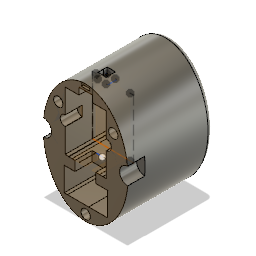
Magnets_Design v1 (Autodesk Fusion 360 design; units mm, degrees)
Autodesk Fusion 360 part; units mm, degrees
note: some values were not read from the file. Set by a fixed rule: which sketch regions a step uses.
(part 1 of 2)
sketch "Sketch1" plane through (0, 0, 0) normal (0, 0, 1) x (1, 0, 0)
  ellipse E0 centre (0, 0) end of major axis (0, 44.45) minor radius 31.75
  line L0 (0, -44.45) -> (0, 44.45)
  line L1 (31.75, 0) -> (-31.75, 0)
extrude "Extrude1" add sketch "Sketch1" along normal blind 63.5
sketch "Sketch2" plane through (0, 0, 63.5) normal (0, 0, 1) x (1, 0, 0)
  ellipse E0 centre (0, 0) end of major axis (0, 44.45) minor radius 31.75
  line L0 (0.1301, 25.8411) -> (10.2901, 25.8411)
  line L1 (0.1301, 25.8411) -> (-10.0299, 25.8411)
  line L2 (-10.0299, 34.8417) -> (-10.0299, -8.8463)
  line L3 (-10.0299, 34.8417) -> (10.4165, 34.8417)
  line L4 (10.4165, 34.8417) -> (10.4165, -8.8757)
  line L5 (10.4165, -8.8757) -> (-10.0299, -8.8463)
  line L6 (0.1933, 34.8417) -> (5.2733, 34.8417)
  line L7 (0.1933, 34.8417) -> (-4.8867, 34.8417)
  line L8 (-4.8867, 34.8417) -> (-4.8867, 39.9217)
  line L9 (-4.8867, 39.9217) -> (5.2733, 39.9217)
  line L10 (5.2733, 39.9217) -> (5.2733, 34.8417)
  dimension "d3" = 10.16
  dimension "d4" = 10.16
  dimension "d5" = 43.688
  dimension "d6" = 5.08
  dimension "d7" = 5.08
  dimension "d8" = 5.08
  measures "d3" distance of E0.centre
  measures "d4" distance of E0.centre
  measures "d6" distance of E0.centre
  measures "d7" distance of E0.centre
extrude "Extrude2" cut sketch "Sketch2" against normal blind 17.78 contours L2 L3 L4 L5 L6 L7 | L3 L6 L7 L8 L9 L10
extrude "Extrude3" cut 1 faces at (1.8866, 5.7066, 45.72) along direction (0, 0, -1) blind 2.54
sketch "Sketch3" plane through (0, 0, 63.5) normal (0, 0, 1) x (1, 0, 0)
  line L0 (10.4165, -8.8757) -> (-10.0299, -8.8463)
  line L1 (-10.0299, -8.8463) -> (-10.0299, 34.8417)
  line L2 (-10.0299, 34.8417) -> (-4.8867, 34.8417)
  line L3 (-4.8867, 34.8417) -> (-4.8867, 39.9217)
  line L4 (-4.8867, 39.9217) -> (5.2733, 39.9217)
  line L5 (5.2733, 39.9217) -> (5.2733, 34.8417)
  line L6 (5.2733, 34.8417) -> (10.4165, 34.8417)
  line L7 (10.4165, 34.8417) -> (10.4165, -8.8757)
  ellipse E0 centre (0, 0) end of major axis (0, 44.45) minor radius 31.75
  line L8 (0.1933, -16.0726) -> (13.7823, -16.0922)
  line L9 (0.1933, -16.0726) -> (-13.3957, -16.053)
  line L10 (13.7823, -16.0922) -> (13.7567, -33.8722)
  line L11 (-13.3957, -16.053) -> (-13.4213, -33.833)
  line L12 (-13.4213, -33.833) -> (13.7567, -33.8722)
  dimension "d13" = 13.589
  dimension "d14" = 13.589
  dimension "d15" = 17.78
  dimension "d16" = 17.78
extrude "Extrude4" cut sketch "Sketch3" against normal blind 53.34 contours L8 L9 L10 L11 L12
sketch "Sketch4" plane through (0, 0, 63.5) normal (0, 0, 1) x (1, 0, 0)
  line L0 (-13.4213, -33.833) -> (-13.3957, -16.053)
  line L1 (-13.3957, -16.053) -> (13.7823, -16.0922)
  line L2 (13.7823, -16.0922) -> (13.7567, -33.8722)
  line L3 (13.7567, -33.8722) -> (-13.4213, -33.833)
  line L4 (10.4165, -8.8757) -> (-10.0299, -8.8463)
  line L5 (-10.0299, -8.8463) -> (-10.0299, 34.8417)
  line L6 (-10.0299, 34.8417) -> (-4.8867, 34.8417)
  line L7 (-4.8867, 34.8417) -> (-4.8867, 39.9217)
  line L8 (-4.8867, 39.9217) -> (5.2733, 39.9217)
  line L9 (5.2733, 39.9217) -> (5.2733, 34.8417)
  line L10 (5.2733, 34.8417) -> (10.4165, 34.8417)
  line L11 (10.4165, 34.8417) -> (10.4165, -8.8757)
  ellipse E0 centre (0, 0) end of major axis (0, 44.45) minor radius 31.75
  line L12 (-4.5003, -8.861) -> (-4.5107, -16.0658)
  line L13 (4.8218, -8.861) -> (4.8114, -16.0792)
  line L14 (-4.5003, -8.861) -> (4.8218, -8.861)
  line L15 (4.8114, -16.0792) -> (-4.5107, -16.0658)
extrude "Extrude5" cut sketch "Sketch4" against normal blind 12.7 contours L1 L4 L12 L13 L14 L15
sketch "Sketch5" plane through (0, 0, 63.5) normal (0, 0, 1) x (1, 0, 0)
  ellipse E0 centre (0, 0) end of major axis (0, 44.45) minor radius 31.75
  line L0 (-4.5107, -16.0658) -> (-4.5003, -8.861)
  line L1 (-4.5003, -8.861) -> (0.1933, -8.861)
  line L2 (0.1933, -8.861) -> (-10.0299, -8.8463)
  line L3 (-10.0299, -8.8463) -> (-10.0299, 34.8417)
  line L4 (-10.0299, 34.8417) -> (-4.8867, 34.8417)
  line L5 (-4.8867, 34.8417) -> (-4.8867, 39.9217)
  line L6 (-4.8867, 39.9217) -> (5.2733, 39.9217)
  line L7 (5.2733, 39.9217) -> (5.2733, 34.8417)
  line L8 (5.2733, 34.8417) -> (10.4165, 34.8417)
  line L9 (10.4165, 34.8417) -> (10.4165, -8.8757)
  line L10 (10.4165, -8.8757) -> (4.8218, -8.8677)
  line L11 (4.8218, -8.8677) -> (4.8114, -16.0792)
  line L12 (4.8114, -16.0792) -> (13.7823, -16.0922)
  line L13 (13.7823, -16.0922) -> (13.7567, -33.8722)
  line L14 (13.7567, -33.8722) -> (-13.4213, -33.833)
  line L15 (-13.4213, -33.833) -> (-13.3957, -16.053)
  line L16 (-13.3957, -16.053) -> (-4.5107, -16.0658)
  circle A0 centre (31.7466, 0.6522) radius 6.35
  circle A1 centre (-31.7467, 0.6454) radius 6.35
  circle A2 centre (-10.0299, 12.9977) radius 6.35
  circle A3 centre (10.4165, 12.983) radius 6.35
  dimension "d21" = 12.7
  dimension "d22" = 12.7
  dimension "d23" = 12.7
  dimension "d24" = 12.7
  measures "d21" diameter of A0
  measures "d22" diameter of A1
  measures "d23" diameter of A2
  measures "d24" diameter of A3
extrude "Extrude6" cut sketch "Sketch5" against normal blind 12.7 contours E0 A1 | E0 A0 | L3 A2 | L9 A3 picked at (-29.7962, -0.9171) picked at (29.729, 2.0886) picked at (-11.8462, 11.3429) picked at (12.7487, 12.3651)
sketch "Sketch6" plane through (0, 0, 63.5) normal (0, 0, 1) x (1, 0, 0)
  arc A0 (-31.4879, -5.6993) -> (-31.3557, 6.9834) centre (-31.7467, 0.6454) ccw
  ellipse E0 centre (0, 0) end of major axis (0, 44.45) minor radius 31.75 (-31.4879, -5.6993) -> (31.4886, -5.6926) ccw
  arc A1 (31.355, 6.9901) -> (31.4886, -5.6926) centre (31.7466, 0.6522) ccw
  ellipse E1 centre (0, 0) end of major axis (0, 44.45) minor radius 31.75 (31.355, 6.9901) -> (-31.3557, 6.9834) ccw
  arc A2 (-10.0299, 19.3477) -> (-10.0299, 6.6477) centre (-10.0299, 12.9977) ccw
  line L0 (-10.0299, 19.3477) -> (-10.0299, 34.8417)
  line L1 (-10.0299, 34.8417) -> (-4.8867, 34.8417)
  line L2 (-4.8867, 34.8417) -> (-4.8867, 39.9217)
  line L3 (-4.8867, 39.9217) -> (5.2733, 39.9217)
  line L4 (5.2733, 39.9217) -> (5.2733, 34.8417)
  line L5 (5.2733, 34.8417) -> (10.4165, 34.8417)
  line L6 (10.4165, 34.8417) -> (10.4165, 19.333)
  arc A3 (10.4165, 6.633) -> (10.4165, 19.333) centre (10.4165, 12.983) ccw
  line L7 (10.4165, 6.633) -> (10.4165, -8.8757)
  line L8 (10.4165, -8.8757) -> (4.8218, -8.8677)
  line L9 (4.8218, -8.8677) -> (4.8114, -16.0792)
  line L10 (4.8114, -16.0792) -> (13.7823, -16.0922)
  line L11 (13.7823, -16.0922) -> (13.7567, -33.8722)
  line L12 (13.7567, -33.8722) -> (-13.4213, -33.833)
  line L13 (-13.4213, -33.833) -> (-13.3957, -16.053)
  line L14 (-13.3957, -16.053) -> (-4.5107, -16.0658)
  line L15 (-4.5107, -16.0658) -> (-4.5003, -8.861)
  line L16 (-4.5003, -8.861) -> (0.1933, -8.861)
  line L17 (0.1933, -8.861) -> (-10.0299, -8.8463)
  line L18 (-10.0299, -8.8463) -> (-10.0299, 6.6477)
  line L19 (22.8671, 20.3792) -> (17.7871, 20.3792)
  line L20 (17.7871, 20.3792) -> (17.7871, 25.4592)
  line L21 (17.7871, 25.4592) -> (22.8671, 25.4592)
  line L22 (22.8671, 25.4592) -> (22.8671, 20.3792)
  line L23 (22.8671, 20.3792) -> (17.7871, 25.4592) construction
  line L24 (17.7871, 20.3792) -> (22.8671, 25.4592) construction
  line L25 (2.5315, -40.6814) -> (-2.5485, -40.6814)
  line L26 (-2.5485, -40.6814) -> (-2.5485, -35.3439)
  line L27 (-2.5485, -35.3439) -> (2.5315, -35.3439)
  line L28 (2.5315, -35.3439) -> (2.5315, -40.6814)
  line L29 (2.5315, -40.6814) -> (-2.5485, -35.3439) construction
  line L30 (-2.5485, -40.6814) -> (2.5315, -35.3439) construction
  line L31 (-17.6615, 20.3792) -> (-22.7415, 20.3792)
  line L32 (-22.7415, 20.3792) -> (-22.7415, 25.4592)
  line L33 (-22.7415, 25.4592) -> (-17.6615, 25.4592)
  line L34 (-17.6615, 25.4592) -> (-17.6615, 20.3792)
  line L35 (-17.6615, 20.3792) -> (-22.7415, 25.4592) construction
  line L36 (-22.7415, 20.3792) -> (-17.6615, 25.4592) construction
  dimension "d27" = 5.08
  dimension "d28" = 5.08
  dimension "d30" = 5.08
  dimension "d31" = 5.08
  dimension "d32" = 5.08
  measures "d28" distance of E0.centre
  measures "d31" distance of E0.centre
extrude "Extrude7" cut sketch "Sketch6" against normal blind 5.08 contours L19 L20 L21 L22 | L25 L26 L27 L28 | L31 L32 L33 L34
sketch "Sketch7" plane through (0, 0, 63.5) normal (0, 0, 1) x (1, 0, 0)
  line L0 (17.7871, 20.3792) -> (17.7871, 25.4592)
  line L1 (17.7871, 25.4592) -> (22.8671, 25.4592)
  line L2 (22.8671, 25.4592) -> (22.8671, 20.3792)
  line L3 (22.8671, 20.3792) -> (17.7871, 20.3792)
  line L4 (-2.5485, -40.6814) -> (-2.5485, -35.3439)
  line L5 (-2.5485, -35.3439) -> (2.5315, -35.3439)
  line L6 (2.5315, -35.3439) -> (2.5315, -40.6814)
  line L7 (2.5315, -40.6814) -> (-2.5485, -40.6814)
  line L8 (-22.7415, 20.3792) -> (-22.7415, 25.4592)
  line L9 (-22.7415, 25.4592) -> (-17.6615, 25.4592)
  line L10 (-17.6615, 25.4592) -> (-17.6615, 20.3792)
  line L11 (-17.6615, 20.3792) -> (-22.7415, 20.3792)
  arc A0 (-31.4879, -5.6993) -> (-31.3557, 6.9834) centre (-31.7467, 0.6454) ccw
  ellipse E0 centre (0, 0) end of major axis (0, 44.45) minor radius 31.75 (-31.4879, -5.6993) -> (31.4886, -5.6926) ccw
  arc A1 (31.355, 6.9901) -> (31.4886, -5.6926) centre (31.7466, 0.6522) ccw
  ellipse E1 centre (0, 0) end of major axis (0, 44.45) minor radius 31.75 (31.355, 6.9901) -> (-31.3557, 6.9834) ccw
  arc A2 (-10.0299, 19.3477) -> (-10.0299, 6.6477) centre (-10.0299, 12.9977) ccw
  line L12 (-10.0299, 19.3477) -> (-10.0299, 34.8417)
  line L13 (-10.0299, 34.8417) -> (-4.8867, 34.8417)
  line L14 (-4.8867, 34.8417) -> (-4.8867, 39.9217)
  line L15 (-4.8867, 39.9217) -> (5.2733, 39.9217)
  line L16 (5.2733, 39.9217) -> (5.2733, 34.8417)
  line L17 (5.2733, 34.8417) -> (10.4165, 34.8417)
  line L18 (10.4165, 34.8417) -> (10.4165, 19.333)
  arc A3 (10.4165, 6.633) -> (10.4165, 19.333) centre (10.4165, 12.983) ccw
  line L19 (10.4165, 6.633) -> (10.4165, -8.8757)
  line L20 (10.4165, -8.8757) -> (4.8218, -8.8677)
  line L21 (4.8218, -8.8677) -> (4.8114, -16.0792)
  line L22 (4.8114, -16.0792) -> (13.7823, -16.0922)
  line L23 (13.7823, -16.0922) -> (13.7567, -33.8722)
  line L24 (13.7567, -33.8722) -> (-13.4213, -33.833)
  line L25 (-13.4213, -33.833) -> (-13.3957, -16.053)
  line L26 (-13.3957, -16.053) -> (-4.5107, -16.0658)
  line L27 (-4.5107, -16.0658) -> (-4.5003, -8.861)
  line L28 (-4.5003, -8.861) -> (0.1933, -8.861)
  line L29 (0.1933, -8.861) -> (-10.0299, -8.8463)
  line L30 (-10.0299, -8.8463) -> (-10.0299, 6.6477)
  line L31 (10.4165, 34.8417) -> (12.9565, 34.8417)
  line L32 (-10.0299, 34.8417) -> (-12.5699, 34.8417)
  line L33 (-12.5699, 34.8417) -> (-12.5699, -8.9534)
  line L34 (-12.5699, -8.9534) -> (-10.0299, -8.8463)
  line L35 (12.9565, 34.8417) -> (12.9565, -8.992)
  line L36 (12.9565, -8.992) -> (10.4165, -8.8757)
  dimension "d36" = 2.54
  dimension "d37" = 2.54
extrude "Extrude8" cut sketch "Sketch7" against normal blind 20.32 contours A2 L12 L32 L33 | A2 L30 L33 L34 | L18 A3 L31 L35 | A3 L19 L35 L36
fillet "Fillet1" radius 3.81 1 edges at (0, -44.45, 0)
sketch "Sketch8" plane through (0, 0, 50.8) normal (0, 0, 1) x (1, 0, 0)
  line L0 (-10.0299, 6.6477) -> (-10.0299, 19.3477)
  arc A0 (-10.0299, 19.3477) -> (-12.5699, 18.8176) centre (-10.0299, 12.9977) ccw
  arc A1 (-12.5699, 18.8176) -> (-12.5699, 7.1778) centre (-10.0299, 12.9977) ccw
  arc A2 (-12.5699, 7.1778) -> (-10.0299, 6.6477) centre (-10.0299, 12.9977) ccw
  line L1 (-12.5699, 18.8176) -> (-12.5699, 7.1778)
  line L2 (12.9565, 18.8029) -> (12.9565, 7.1631)
  line L3 (12.9565, 18.8029) -> (12.9565, 7.1631)
extrude "Extrude9" cut sketch "Sketch8" against normal blind 7.62 contours L0 A0 A2 L1
sketch "Sketch9" plane through (0, 0, 50.8) normal (0, 0, 1) x (1, 0, 0)
  arc A0 (12.9565, 18.8029) -> (10.4165, 19.333) centre (10.4165, 12.983) ccw
  line L0 (10.4165, 19.333) -> (10.4165, 6.633)
  arc A1 (10.4165, 6.633) -> (12.9565, 7.1631) centre (10.4165, 12.983) ccw
  arc A2 (12.9565, 7.1631) -> (12.9565, 18.8029) centre (10.4165, 12.983) ccw
  line L1 (12.9565, 18.8029) -> (12.9565, 7.1631)
extrude "Extrude10" cut sketch "Sketch9" against normal blind 7.62 contours A0 L0 A1 L1
sketch "Sketch10" plane through (-0.0128, -8.8607, 0) normal (0.001441, 0.999999, 0) x (0, 0, -1)
  line L0 (-63.5, -0.2061) -> (-50.8, -0.2061)
  line L1 (-50.8, -0.2061) -> (-50.8, -4.8345)
  line L2 (-50.8, -4.8345) -> (-63.5, -4.8345)
  line L3 (-63.5, -4.8345) -> (-63.5, -10.4293)
  line L4 (-63.5, -10.4293) -> (-43.18, -10.4293)
  line L5 (-43.18, -10.4293) -> (-43.18, 10.0172)
  line L6 (-43.18, 10.0172) -> (-63.5, 10.0172)
  line L7 (-63.5, 10.0172) -> (-63.5, -0.2061)
  line L8 (-63.5, 4.9056) -> (-50.7412, 4.9056)
  line L9 (-51.1674, -0.2061) -> (-50.7412, 4.9056)
extrude "Extrude11" add 1 faces at (0.1647, -13.6687, 50.8) along direction (0, 0, 1) blind 12.7
sketch "Sketch11" plane through (0, 0, 63.5) normal (0, 0, 1) x (1, 0, 0)
  line L0 (-13.3957, -16.053) -> (13.7823, -16.0922)
  line L1 (13.7823, -16.0922) -> (13.7567, -33.8722)
  line L2 (13.7567, -33.8722) -> (-13.4213, -33.833)
  line L3 (-13.4213, -33.833) -> (-13.3957, -16.053)
  arc A0 (-31.4879, -5.6993) -> (-31.3557, 6.9834) centre (-31.7467, 0.6454) ccw
  ellipse E0 centre (0, 0) end of major axis (0, 44.45) minor radius 31.75 (-31.4879, -5.6993) -> (31.4886, -5.6926) ccw
  arc A1 (31.355, 6.9901) -> (31.4886, -5.6926) centre (31.7466, 0.6522) ccw
  ellipse E1 centre (0, 0) end of major axis (0, 44.45) minor radius 31.75 (31.355, 6.9901) -> (-31.3557, 6.9834) ccw
  line L4 (-22.7415, 20.3792) -> (-22.7415, 25.4592)
  line L5 (-22.7415, 25.4592) -> (-17.6615, 25.4592)
  line L6 (-17.6615, 25.4592) -> (-17.6615, 20.3792)
  line L7 (-17.6615, 20.3792) -> (-22.7415, 20.3792)
  line L8 (-2.5485, -40.6814) -> (-2.5485, -35.3439)
  line L9 (-2.5485, -35.3439) -> (2.5315, -35.3439)
  line L10 (2.5315, -35.3439) -> (2.5315, -40.6814)
  line L11 (2.5315, -40.6814) -> (-2.5485, -40.6814)
  line L12 (17.7871, 20.3792) -> (17.7871, 25.4592)
  line L13 (17.7871, 25.4592) -> (22.8671, 25.4592)
  line L14 (22.8671, 25.4592) -> (22.8671, 20.3792)
  line L15 (22.8671, 20.3792) -> (17.7871, 20.3792)
  line L16 (10.4165, -8.8757) -> (-10.0299, -8.8463)
  line L17 (-10.0299, -8.8463) -> (-12.5699, -8.9534)
  line L18 (-12.5699, -8.9534) -> (-12.5699, 7.1778)
  arc A2 (-12.5699, 18.8176) -> (-12.5699, 7.1778) centre (-10.0299, 12.9977) ccw
  line L19 (-12.5699, 18.8176) -> (-12.5699, 34.8417)
  line L20 (-12.5699, 34.8417) -> (-4.8867, 34.8417)
  line L21 (-4.8867, 34.8417) -> (-4.8867, 39.9217)
  line L22 (-4.8867, 39.9217) -> (5.2733, 39.9217)
  line L23 (5.2733, 39.9217) -> (5.2733, 34.8417)
  line L24 (5.2733, 34.8417) -> (12.9565, 34.8417)
  line L25 (12.9565, 34.8417) -> (12.9565, 18.8029)
  arc A3 (12.9565, 7.1631) -> (12.9565, 18.8029) centre (10.4165, 12.983) ccw
  line L26 (12.9565, 7.1631) -> (12.9565, -8.992)
  line L27 (12.9565, -8.992) -> (10.4165, -8.8757)
  line L28 (-7.8564, -8.8494) -> (-7.8668, -16.061)
  line L29 (4.8218, -8.8677) -> (10.4165, -8.8757)
  line L30 (7.6191, -8.8717) -> (7.6088, -16.0833)
  line L31 (-7.8668, -16.061) -> (7.6088, -16.0833)
  line L32 (7.6191, -8.8717) -> (-7.8564, -8.8494)
extrude "Extrude12" cut sketch "Sketch11" against normal blind 12.7 contours L0 L16 L28 L29 L30 L31 L32
sketch "Sketch12" plane through (0, 0, 43.18) normal (0, 0, 1) x (1, 0, 0)
  line L0 (-10.0299, -8.8463) -> (10.4165, -8.8757)
  line L1 (10.4165, -8.8757) -> (12.9565, -8.992)
  line L2 (12.9565, -8.992) -> (12.9565, 34.8417)
  line L3 (12.9565, 34.8417) -> (5.2733, 34.8417)
  line L4 (5.2733, 34.8417) -> (5.2733, 39.9217)
  line L5 (5.2733, 39.9217) -> (-4.8867, 39.9217)
  line L6 (-4.8867, 39.9217) -> (-4.8867, 34.8417)
  line L7 (-4.8867, 34.8417) -> (-12.5699, 34.8417)
  line L8 (-12.5699, 34.8417) -> (-12.5699, -8.9534)
  line L9 (-12.5699, -8.9534) -> (-10.0299, -8.8463)
  line L10 (-12.5699, 34.8417) -> (-15.1099, 34.8417) construction
  line L11 (12.9565, 34.8417) -> (15.4965, 34.8417) construction
  line L12 (-15.1099, 34.8417) -> (-15.1099, -8.6009) construction
  line L13 (-15.1099, -8.6009) -> (12.9565, -8.992) construction
  line L14 (15.4965, 34.8417) -> (15.4965, -8.992) construction
  line L15 (15.4965, -8.992) -> (-15.1099, -8.6009) construction
  line L16 (-15.1099, -8.6009) -> (-15.1099, 34.8417) construction
  line L17 (12.9565, 34.8417) -> (15.4965, 34.8417) construction
  dimension "d48" = 2.54
  dimension "d49" = 2.54
sketch "Sketch13" plane through (0, 0, 63.5) normal (0, 0, 1) x (1, 0, 0)
  line L0 (7.6191, -8.8717) -> (7.6088, -16.0833)
  line L1 (7.6088, -16.0833) -> (13.7823, -16.0922)
  line L2 (13.7823, -16.0922) -> (13.7567, -33.8722)
  line L3 (13.7567, -33.8722) -> (-13.4213, -33.833)
  line L4 (-13.4213, -33.833) -> (-13.3957, -16.053)
  line L5 (-13.3957, -16.053) -> (-7.8668, -16.061)
  line L6 (-7.8668, -16.061) -> (-7.8564, -8.8494)
  line L7 (-7.8564, -8.8494) -> (-10.0299, -8.8463)
  line L8 (-10.0299, -8.8463) -> (-12.5699, -8.9534)
  line L9 (-12.5699, -8.9534) -> (-12.5699, 7.1778)
  arc A0 (-12.5699, 18.8176) -> (-12.5699, 7.1778) centre (-10.0299, 12.9977) ccw
  line L10 (-12.5699, 18.8176) -> (-12.5699, 34.8417)
  line L11 (-12.5699, 34.8417) -> (-4.8867, 34.8417)
  line L12 (-4.8867, 34.8417) -> (-4.8867, 39.9217)
  line L13 (-4.8867, 39.9217) -> (5.2733, 39.9217)
  line L14 (5.2733, 39.9217) -> (5.2733, 34.8417)
  line L15 (5.2733, 34.8417) -> (12.9565, 34.8417)
  line L16 (12.9565, 34.8417) -> (12.9565, 18.8029)
  arc A1 (12.9565, 7.1631) -> (12.9565, 18.8029) centre (10.4165, 12.983) ccw
  line L17 (12.9565, 7.1631) -> (12.9565, -8.992)
  line L18 (12.9565, -8.992) -> (10.4165, -8.8757)
  line L19 (10.4165, -8.8757) -> (7.6191, -8.8717)
  arc A2 (-31.4879, -5.6993) -> (-31.3557, 6.9834) centre (-31.7467, 0.6454) ccw
  ellipse E0 centre (0, 0) end of major axis (0, 44.45) minor radius 31.75 (-31.4879, -5.6993) -> (31.4886, -5.6926) ccw
  arc A3 (31.355, 6.9901) -> (31.4886, -5.6926) centre (31.7466, 0.6522) ccw
  ellipse E1 centre (0, 0) end of major axis (0, 44.45) minor radius 31.75 (31.355, 6.9901) -> (-31.3557, 6.9834) ccw
  line L20 (-22.7415, 20.3792) -> (-22.7415, 25.4592)
  line L21 (-22.7415, 25.4592) -> (-17.6615, 25.4592)
  line L22 (-17.6615, 25.4592) -> (-17.6615, 20.3792)
  line L23 (-17.6615, 20.3792) -> (-22.7415, 20.3792)
  line L24 (-2.5485, -40.6814) -> (-2.5485, -35.3439)
  line L25 (-2.5485, -35.3439) -> (2.5315, -35.3439)
  line L26 (2.5315, -35.3439) -> (2.5315, -40.6814)
  line L27 (2.5315, -40.6814) -> (-2.5485, -40.6814)
  line L28 (17.7871, 20.3792) -> (17.7871, 25.4592)
  line L29 (17.7871, 25.4592) -> (22.8671, 25.4592)
  line L30 (22.8671, 25.4592) -> (22.8671, 20.3792)
  line L31 (22.8671, 20.3792) -> (17.7871, 20.3792)
  line L32 (12.9565, 34.8417) -> (15.4965, 34.8417)
  line L33 (15.4965, 34.8417) -> (15.4965, -8.992)
  line L34 (15.4965, -8.992) -> (-15.1099, -8.6009)
  line L35 (-15.1099, -8.6009) -> (-15.1099, 34.8417)
  line L36 (-15.1099, 34.8417) -> (15.4965, 34.8417)
extrude "Extrude13" cut sketch "Sketch13" against normal blind 17.78 contours L0 L9 A0 L10 L11 L15 L16 A1 L17 L18 L19 L33 L34 L35 L36 | L9 A0 L34 L35 | A1 L17 L33 L34 | A0 L10 L35 L36 | L16 A1 L32 L33 L36
extrude "Extrude14" cut 2 faces at (-13.4166, 5.8692, 45.72) (14.6499, 5.6301, 45.72) along direction (0, 0, -1) blind 2.54
sketch "Sketch14" plane through (0, 0, 50.8) normal (0, 0, 1) x (1, 0, 0)
  line L0 (-15.1099, 9.1877) -> (-15.1099, 16.8077)
  arc A0 (-15.1099, 16.8077) -> (-15.1099, 9.1877) centre (-10.0299, 12.9977) ccw
sketch "Sketch15" plane through (0, 0, 63.5) normal (0, 0, 1) x (1, 0, 0)
  line L0 (17.7871, 20.3792) -> (17.7871, 25.4592)
  line L1 (17.7871, 25.4592) -> (22.8671, 25.4592)
  line L2 (22.8671, 25.4592) -> (22.8671, 20.3792)
  line L3 (22.8671, 20.3792) -> (17.7871, 20.3792)
  line L4 (-2.5485, -40.6814) -> (-2.5485, -35.3439)
  line L5 (-2.5485, -35.3439) -> (2.5315, -35.3439)
  line L6 (2.5315, -35.3439) -> (2.5315, -40.6814)
  line L7 (2.5315, -40.6814) -> (-2.5485, -40.6814)
  line L8 (-22.7415, 20.3792) -> (-22.7415, 25.4592)
  line L9 (-22.7415, 25.4592) -> (-17.6615, 25.4592)
  line L10 (-17.6615, 25.4592) -> (-17.6615, 20.3792)
  line L11 (-17.6615, 20.3792) -> (-22.7415, 20.3792)
  arc A0 (-31.4879, -5.6993) -> (-31.3557, 6.9834) centre (-31.7467, 0.6454) ccw
  ellipse E0 centre (0, 0) end of major axis (0, 44.45) minor radius 31.75 (-31.4879, -5.6993) -> (31.4886, -5.6926) ccw
  arc A1 (31.355, 6.9901) -> (31.4886, -5.6926) centre (31.7466, 0.6522) ccw
  ellipse E1 centre (0, 0) end of major axis (0, 44.45) minor radius 31.75 (31.355, 6.9901) -> (-31.3557, 6.9834) ccw
  line L12 (15.4965, 9.173) -> (15.4965, -8.992)
  line L13 (15.4965, -8.992) -> (12.9565, -8.9595)
  line L14 (12.9565, -8.9595) -> (12.9565, -8.992)
  line L15 (12.9565, -8.992) -> (10.4165, -8.8757)
  line L16 (10.4165, -8.8757) -> (7.6191, -8.8717)
  line L17 (7.6191, -8.8717) -> (7.6088, -16.0833)
  line L18 (7.6088, -16.0833) -> (13.7823, -16.0922)
  line L19 (13.7823, -16.0922) -> (13.7567, -33.8722)
  line L20 (13.7567, -33.8722) -> (-13.4213, -33.833)
  line L21 (-13.4213, -33.833) -> (-13.3957, -16.053)
  line L22 (-13.3957, -16.053) -> (-7.8668, -16.061)
  line L23 (-7.8668, -16.061) -> (-7.8564, -8.8494)
  line L24 (-7.8564, -8.8494) -> (-10.0299, -8.8463)
  line L25 (-10.0299, -8.8463) -> (-12.5699, -8.9534)
  line L26 (-12.5699, -8.9534) -> (-12.5699, -8.6333)
  line L27 (-12.5699, -8.6333) -> (-15.1099, -8.6009)
  line L28 (-15.1099, -8.6009) -> (-15.1099, 9.1877)
  arc A2 (-15.1099, 16.8077) -> (-15.1099, 9.1877) centre (-10.0299, 12.9977) ccw
  line L29 (-15.1099, 16.8077) -> (-15.1099, 34.8417)
  line L30 (-15.1099, 34.8417) -> (-4.8867, 34.8417)
  line L31 (-4.8867, 34.8417) -> (-4.8867, 39.9217)
  line L32 (-4.8867, 39.9217) -> (5.2733, 39.9217)
  line L33 (5.2733, 39.9217) -> (5.2733, 34.8417)
  line L34 (5.2733, 34.8417) -> (15.4965, 34.8417)
  line L35 (15.4965, 34.8417) -> (15.4965, 16.793)
  arc A3 (15.4965, 9.173) -> (15.4965, 16.793) centre (10.4165, 12.983) ccw
  circle A4 centre (-15.1099, 13.1204) radius 3.81
  line L36 (-15.1099, -8.6009) -> (-15.1099, 34.8417)
  circle A5 centre (15.4965, 12.983) radius 3.8115
  line L37 (15.4965, 16.793) -> (15.4965, 9.173)
  dimension "d54" = 7.62
  measures "d54" diameter of A4
extrude "Extrude15" cut sketch "Sketch15" against normal blind 12.7 contours A3 L37 | A3 A5 | A2 L29 A4 L36 | A2 A4 L36 picked at (-15.2709, 14.0593)
sketch "Sketch16" plane through (0, 0, 63.5) normal (0, 0, 1) x (1, 0, 0)
  arc A0 (-15.1099, 16.9304) -> (-15.2005, 9.3115) centre (-15.1099, 13.1204) ccw
  line L0 (-15.1099, 16.9304) -> (-15.1099, 34.8417)
  line L1 (-15.1099, 34.8417) -> (-4.8867, 34.8417)
  line L2 (-4.8867, 34.8417) -> (-4.8867, 39.9217)
  line L3 (-4.8867, 39.9217) -> (5.2733, 39.9217)
  line L4 (5.2733, 39.9217) -> (5.2733, 34.8417)
  line L5 (5.2733, 34.8417) -> (15.4965, 34.8417)
  line L6 (15.4965, 34.8417) -> (15.4965, 16.7945)
  arc A1 (15.4965, 9.1715) -> (15.4965, 16.7945) centre (15.4965, 12.983) ccw
  line L7 (15.4965, 9.1715) -> (15.4965, -8.992)
  line L8 (15.4965, -8.992) -> (12.9565, -8.9595)
  line L9 (12.9565, -8.9595) -> (12.9565, -8.992)
  line L10 (12.9565, -8.992) -> (10.4165, -8.8757)
  line L11 (10.4165, -8.8757) -> (7.6191, -8.8717)
  line L12 (7.6191, -8.8717) -> (7.6088, -16.0833)
  line L13 (7.6088, -16.0833) -> (13.7823, -16.0922)
  line L14 (13.7823, -16.0922) -> (13.7567, -33.8722)
  line L15 (13.7567, -33.8722) -> (-13.4213, -33.833)
  line L16 (-13.4213, -33.833) -> (-13.3957, -16.053)
  line L17 (-13.3957, -16.053) -> (-7.8668, -16.061)
  line L18 (-7.8668, -16.061) -> (-7.8564, -8.8494)
  line L19 (-7.8564, -8.8494) -> (-10.0299, -8.8463)
  line L20 (-10.0299, -8.8463) -> (-12.5699, -8.9534)
  line L21 (-12.5699, -8.9534) -> (-12.5699, -8.6333)
  line L22 (-12.5699, -8.6333) -> (-15.1099, -8.6009)
  line L23 (-15.1099, -8.6009) -> (-15.1099, 9.1877)
  arc A2 (-15.2005, 9.3115) -> (-15.1099, 9.1877) centre (-10.0299, 12.9977) ccw
  line L24 (17.7871, 20.3792) -> (17.7871, 25.4592)
  line L25 (17.7871, 25.4592) -> (22.8671, 25.4592)
  line L26 (22.8671, 25.4592) -> (22.8671, 20.3792)
  line L27 (22.8671, 20.3792) -> (17.7871, 20.3792)
  line L28 (-2.5485, -40.6814) -> (-2.5485, -35.3439)
  line L29 (-2.5485, -35.3439) -> (2.5315, -35.3439)
  line L30 (2.5315, -35.3439) -> (2.5315, -40.6814)
  line L31 (2.5315, -40.6814) -> (-2.5485, -40.6814)
  line L32 (-22.7415, 20.3792) -> (-22.7415, 25.4592)
  line L33 (-22.7415, 25.4592) -> (-17.6615, 25.4592)
  line L34 (-17.6615, 25.4592) -> (-17.6615, 20.3792)
  line L35 (-17.6615, 20.3792) -> (-22.7415, 20.3792)
  arc A3 (-31.4879, -5.6993) -> (-31.3557, 6.9834) centre (-31.7467, 0.6454) ccw
  ellipse E0 centre (0, 0) end of major axis (0, 44.45) minor radius 31.75 (-31.4879, -5.6993) -> (31.4886, -5.6926) ccw
  arc A4 (31.355, 6.9901) -> (31.4886, -5.6926) centre (31.7466, 0.6522) ccw
  ellipse E1 centre (0, 0) end of major axis (0, 44.45) minor radius 31.75 (31.355, 6.9901) -> (-31.3557, 6.9834) ccw
  line L36 (-13.3957, -16.053) -> (-15.9357, -16.053)
  line L37 (-15.9357, -16.053) -> (-15.9357, -33.833)
  line L38 (-15.9357, -33.833) -> (-13.3957, -33.833)
  line L39 (-13.3957, -33.833) -> (-13.3957, -16.053)
  line L40 (13.7823, -16.0922) -> (16.3223, -16.0922)
  line L41 (16.3223, -16.0922) -> (16.3223, -33.8722)
  line L42 (16.3223, -33.8722) -> (13.7823, -33.8722)
  line L43 (13.7823, -33.8722) -> (13.7823, -16.0922)
  line L44 (-7.8668, -16.061) -> (7.6088, -16.0833)
  line L45 (-15.9357, -16.053) -> (16.3223, -16.053)
  line L46 (16.3223, -16.053) -> (16.3223, -16.0922)
  line L47 (16.3223, -16.0922) -> (-15.9357, -16.0922)
  line L48 (-15.9357, -16.0922) -> (-15.9357, -16.053)
  line L49 (16.3223, -33.8722) -> (-15.9357, -33.8722)
  line L50 (-15.9357, -33.8722) -> (-15.9357, -33.833)
  line L51 (-15.9357, -33.833) -> (16.3223, -33.833)
  line L52 (16.3223, -33.833) -> (16.3223, -33.8722)
  dimension "d57" = 2.54
  dimension "d58" = 17.78
  dimension "d59" = 2.54
  dimension "d60" = 17.78
extrude "Extrude16" cut sketch "Sketch16" against normal blind 53.34 contours L14 L39 L47 L51 | L16 L37 L38 L47 L51 | L40 L41 L43 L47 L51
extrude "Extrude17" add 1 faces at (13.7737, -22.0188, 45.72) along direction (-0.999999, 0.001441, 0) blind 11.43
sketch "Sketch17" plane through (0, 0, 63.5) normal (0, 0, 1) x (1, 0, 0)
  line L0 (13.7823, -16.0922) -> (16.3223, -16.0922)
  line L1 (16.3223, -16.0922) -> (16.3223, -33.833)
  line L2 (16.3223, -33.833) -> (13.7823, -33.833)
  line L3 (13.7823, -33.833) -> (13.7823, -16.0922)
  arc A0 (-31.4879, -5.6993) -> (-31.3557, 6.9834) centre (-31.7467, 0.6454) ccw
  ellipse E0 centre (0, 0) end of major axis (0, 44.45) minor radius 31.75 (-31.4879, -5.6993) -> (31.4886, -5.6926) ccw
  arc A1 (31.355, 6.9901) -> (31.4886, -5.6926) centre (31.7466, 0.6522) ccw
  ellipse E1 centre (0, 0) end of major axis (0, 44.45) minor radius 31.75 (31.355, 6.9901) -> (-31.3557, 6.9834) ccw
  line L4 (-22.7415, 20.3792) -> (-22.7415, 25.4592)
  line L5 (-22.7415, 25.4592) -> (-17.6615, 25.4592)
  line L6 (-17.6615, 25.4592) -> (-17.6615, 20.3792)
  line L7 (-17.6615, 20.3792) -> (-22.7415, 20.3792)
  line L8 (-2.5485, -40.6814) -> (-2.5485, -35.3439)
  line L9 (-2.5485, -35.3439) -> (2.5315, -35.3439)
  line L10 (2.5315, -35.3439) -> (2.5315, -40.6814)
  line L11 (2.5315, -40.6814) -> (-2.5485, -40.6814)
  line L12 (17.7871, 20.3792) -> (17.7871, 25.4592)
  line L13 (17.7871, 25.4592) -> (22.8671, 25.4592)
  line L14 (22.8671, 25.4592) -> (22.8671, 20.3792)
  line L15 (22.8671, 20.3792) -> (17.7871, 20.3792)
  line L16 (7.6088, -16.0833) -> (2.3523, -16.0757)
  line L17 (2.3523, -16.0757) -> (2.3267, -33.8557)
  line L18 (2.3267, -33.8557) -> (-13.4085, -33.833)
  line L19 (-13.4085, -33.833) -> (-15.9357, -33.833)
  line L20 (-15.9357, -33.833) -> (-15.9357, -16.0922)
  line L21 (-15.9357, -16.0922) -> (-13.3958, -16.0922)
  line L22 (-13.3958, -16.0922) -> (-13.3957, -16.053)
  line L23 (-13.3957, -16.053) -> (-7.8668, -16.061)
  line L24 (-7.8668, -16.061) -> (-7.8564, -8.8494)
  line L25 (-7.8564, -8.8494) -> (-10.0299, -8.8463)
  line L26 (-10.0299, -8.8463) -> (-12.5699, -8.9534)
  line L27 (-12.5699, -8.9534) -> (-12.5699, -8.6333)
  line L28 (-12.5699, -8.6333) -> (-15.1099, -8.6009)
  line L29 (-15.1099, -8.6009) -> (-15.1099, 9.1877)
  arc A2 (-15.2005, 9.3115) -> (-15.1099, 9.1877) centre (-10.0299, 12.9977) ccw
  arc A3 (-15.1099, 16.9304) -> (-15.2005, 9.3115) centre (-15.1099, 13.1204) ccw
  line L30 (-15.1099, 16.9304) -> (-15.1099, 34.8417)
  line L31 (-15.1099, 34.8417) -> (-4.8867, 34.8417)
  line L32 (-4.8867, 34.8417) -> (-4.8867, 39.9217)
  line L33 (-4.8867, 39.9217) -> (5.2733, 39.9217)
  line L34 (5.2733, 39.9217) -> (5.2733, 34.8417)
  line L35 (5.2733, 34.8417) -> (15.4965, 34.8417)
  line L36 (15.4965, 34.8417) -> (15.4965, 16.7945)
  arc A4 (15.4965, 9.1715) -> (15.4965, 16.7945) centre (15.4965, 12.983) ccw
  line L37 (15.4965, 9.1715) -> (15.4965, -8.992)
  line L38 (15.4965, -8.992) -> (12.9565, -8.9595)
  line L39 (12.9565, -8.9595) -> (12.9565, -8.992)
  line L40 (12.9565, -8.992) -> (10.4165, -8.8757)
  line L41 (10.4165, -8.8757) -> (7.6191, -8.8717)
  line L42 (7.6191, -8.8717) -> (7.6088, -16.0833)
  line L43 (2.3523, -16.0757) -> (16.3223, -16.0922)
  line L44 (16.3223, -33.833) -> (2.3267, -33.8557)
extrude "Extrude18" cut sketch "Sketch17" against normal blind 53.34 contours L0 L2 L3 L16 L17 L43 L44 | L0 L1 L2 L3
sketch "Sketch18" plane through (0, 0, 63.5) normal (0, 0, 1) x (1, 0, 0)
  line L0 (17.7871, 20.3792) -> (17.7871, 25.4592)
  line L1 (17.7871, 25.4592) -> (22.8671, 25.4592)
  line L2 (22.8671, 25.4592) -> (22.8671, 20.3792)
  line L3 (22.8671, 20.3792) -> (17.7871, 20.3792)
  line L4 (-2.5485, -40.6814) -> (-2.5485, -35.3439)
  line L5 (-2.5485, -35.3439) -> (2.5315, -35.3439)
  line L6 (2.5315, -35.3439) -> (2.5315, -40.6814)
  line L7 (2.5315, -40.6814) -> (-2.5485, -40.6814)
  line L8 (-22.7415, 20.3792) -> (-22.7415, 25.4592)
  line L9 (-22.7415, 25.4592) -> (-17.6615, 25.4592)
  line L10 (-17.6615, 25.4592) -> (-17.6615, 20.3792)
  line L11 (-17.6615, 20.3792) -> (-22.7415, 20.3792)
  arc A0 (-31.4879, -5.6993) -> (-31.3557, 6.9834) centre (-31.7467, 0.6454) ccw
  ellipse E0 centre (0, 0) end of major axis (0, 44.45) minor radius 31.75 (-31.4879, -5.6993) -> (31.4886, -5.6926) ccw
  arc A1 (31.355, 6.9901) -> (31.4886, -5.6926) centre (31.7466, 0.6522) ccw
  ellipse E1 centre (0, 0) end of major axis (0, 44.45) minor radius 31.75 (31.355, 6.9901) -> (-31.3557, 6.9834) ccw
  line L12 (7.6088, -16.0819) -> (16.3223, -16.0922)
  line L13 (16.3223, -16.0922) -> (16.3223, -33.833)
  line L14 (16.3223, -33.833) -> (2.3267, -33.8557)
  line L15 (2.3267, -33.8557) -> (-13.4085, -33.833)
  line L16 (-13.4085, -33.833) -> (-15.9357, -33.833)
  line L17 (-15.9357, -33.833) -> (-15.9357, -16.0922)
  line L18 (-15.9357, -16.0922) -> (-13.3958, -16.0922)
  line L19 (-13.3958, -16.0922) -> (-13.3957, -16.053)
  line L20 (-13.3957, -16.053) -> (-7.8668, -16.061)
  line L21 (-7.8668, -16.061) -> (-7.8564, -8.8494)
  line L22 (-7.8564, -8.8494) -> (-10.0299, -8.8463)
  line L23 (-10.0299, -8.8463) -> (-12.5699, -8.9534)
  line L24 (-12.5699, -8.9534) -> (-12.5699, -8.6333)
  line L25 (-12.5699, -8.6333) -> (-15.1099, -8.6009)
  line L26 (-15.1099, -8.6009) -> (-15.1099, 9.1877)
  arc A2 (-15.2005, 9.3115) -> (-15.1099, 9.1877) centre (-10.0299, 12.9977) ccw
  arc A3 (-15.1099, 16.9304) -> (-15.2005, 9.3115) centre (-15.1099, 13.1204) ccw
  line L27 (-15.1099, 16.9304) -> (-15.1099, 34.8417)
  line L28 (-15.1099, 34.8417) -> (-4.8867, 34.8417)
  line L29 (-4.8867, 34.8417) -> (-4.8867, 39.9217)
  line L30 (-4.8867, 39.9217) -> (5.2733, 39.9217)
  line L31 (5.2733, 39.9217) -> (5.2733, 34.8417)
  line L32 (5.2733, 34.8417) -> (15.4965, 34.8417)
  line L33 (15.4965, 34.8417) -> (15.4965, 16.7945)
  arc A4 (15.4965, 9.1715) -> (15.4965, 16.7945) centre (15.4965, 12.983) ccw
  line L34 (15.4965, 9.1715) -> (15.4965, -8.992)
  line L35 (15.4965, -8.992) -> (12.9565, -8.9595)
  line L36 (12.9565, -8.9595) -> (12.9565, -8.992)
  line L37 (12.9565, -8.992) -> (10.4165, -8.8757)
  line L38 (10.4165, -8.8757) -> (7.6191, -8.8717)
  line L39 (7.6191, -8.8717) -> (7.6088, -16.0819)
  spline S0 degree 3 poles (0, -44.45) (-1.3864, -44.45) (-2.7724, -44.3217) (-5.5257, -43.816) (-6.8908, -43.4322) (-11.0228, -41.8851) (-13.5882, -40.3391) (-17.8123, -36.9324) (-19.5534, -35.139) (-22.6333, -31.3062) (-23.9736, -29.2654) (-27.9565, -22.0369) (-29.77, -16.5059) (-31.65, -6.0775) (-31.9288, -1.1924) (-31.4054, 7.6683) (-30.7828, 11.6568) (-28.7725, 19.1897) (-27.4407, 22.7479) (-23.9024, 29.5631) (-21.6837, 32.824) (-17.5156, 37.1551) (-15.9665, 38.5126) (-11.7153, 41.5067) (-8.807, 42.9389) (-2.7928, 44.466) (0.2642, 44.6422) (6.5099, 43.7518) (9.6437, 42.5582) (16.2066, 38.6571) (19.3342, 35.5962) (24.4061, 28.85) (26.3669, 25.1457) (29.8026, 16.3398) (30.9688, 11.137) (31.7703, 2.7462) (31.8289, -0.4177) (31.4051, -7.7792) (30.7371, -11.9702) (28.892, -18.637) (27.9933, -21.1745) (25.6386, -26.4241) (24.1257, -29.118) (20.8447, -33.6511) (19.1878, -35.5537) (15.4585, -38.9479) (13.3908, -40.4473) (9.0457, -42.7192) (6.8043, -43.5433) (2.9997, -44.2995) (1.5001, -44.45) (0, -44.45) knots -3.141593 -3.141593 -3.141593 -3.141593 -3.041454 -3.041454 -2.938441 -2.938441 -2.717035 -2.717035 -2.524692 -2.524692 -2.33235 -2.33235 -1.867558 -1.867558 -1.471204 -1.471204 -1.144306 -1.144306 -0.83981 -0.83981 -0.531541 -0.531541 -0.374414 -0.374414 -0.138256 -0.138256 0.077774 0.077774 0.318781 0.318781 0.6499 0.6499 0.981415 0.981415 1.410535 1.410535 1.667861 1.667861 2.011337 2.011337 2.227869 2.227869 2.472577 2.472577 2.668087 2.668087 2.859878 2.859878 3.033241 3.033241 3.141593 3.141593 3.141593 3.141593
  line L40 (0.1933, 39.9217) -> (0.1933, 44.4452)
  line L41 (-4.8867, 39.9217) -> (-4.8867, 43.9204)
  line L42 (5.2733, 39.9217) -> (5.2733, 43.8326)
  line L43 (-4.8867, 41.3657) -> (5.2733, 41.3657)
  line L44 (-4.8867, 43.0743) -> (5.2733, 43.0743)
extrude "Extrude19" cut sketch "Sketch18" against normal blind 17.78 contours L40 L41 L43 L44 | L40 L42 L43 L44
ref_plane "WorkPlane1" through (-0.0469, 0.0803, 31.75) normal (0, 0, -1) x (-1, 0, 0)
sketch "Sketch19" plane through (-0.0469, 0.0803, 31.75) normal (0, 0, -1) x (1, 0, 0)
sketch "Sketch20" plane through (0, 39.9217, 0) normal (0, -1, 0) x (1, 0, 0)
  line L0 (5.2733, 63.5) -> (-4.8867, 63.5)
  line L1 (-4.8867, 63.5) -> (-4.8867, 43.18)
  line L2 (-4.8867, 43.18) -> (5.2733, 43.18)
  line L3 (5.2733, 43.18) -> (5.2733, 63.5)
  line L4 (0, 43.18) -> (0, 44.45)
  line L5 (0, 43.18) -> (0, 44.45)
  line L6 (0, 44.45) -> (0, 46.99)
  line L7 (0, 46.99) -> (3.0833, 46.99)
  line L8 (0, 44.45) -> (3.11, 44.45)
  line L9 (3.11, 44.45) -> (3.0833, 46.99)
  line L10 (0, 44.45) -> (-3.0988, 44.45)
  line L11 (-3.0988, 44.45) -> (-3.0988, 46.9504)
  line L12 (0, 46.99) -> (-3.0988, 46.9504)
  dimension "d69" = 1.27
  dimension "d70" = 1.27
  dimension "d71" = 2.54
  dimension "d72" = 3.0988
  measures "d69" distance of origin
extrude "Extrude20" cut sketch "Sketch20" against normal blind 22.86 contours L6 L10 L11 L12 | L6 L7 L8 L9
extrude "Extrude21" add 2 faces at (3.8222, 42.5048, 45.72) (-4.2907, 42.5048, 45.72) along direction (0, 0, 1) blind 17.78
sketch "Sketch21" plane through (0, 39.9217, 0) normal (0, -1, 0) x (1, 0, 0)
  line L0 (3.0833, 46.99) -> (3.11, 44.45)
  line L1 (3.11, 44.45) -> (-3.0988, 44.45)
  line L2 (-3.0988, 44.45) -> (-3.0988, 46.9504)
  line L3 (-3.0988, 46.9504) -> (0, 46.99)
  line L4 (0, 46.99) -> (3.0833, 46.99)
  line L5 (5.2733, 63.5) -> (-4.8867, 63.5)
  line L6 (-4.8867, 63.5) -> (-4.8867, 43.18)
  line L7 (-4.8867, 43.18) -> (5.2733, 43.18)
  line L8 (5.2733, 43.18) -> (5.2733, 63.5)
  line L9 (-3.0988, 46.9504) -> (-3.1539, 51.2681)
  line L10 (3.0833, 46.99) -> (3.0833, 51.308)
  line L11 (-3.1539, 51.2681) -> (3.0833, 51.308)
  dimension "d77" = 4.318
  dimension "d78" = 4.318
extrude "Extrude22" cut sketch "Sketch21" against normal blind 35.56 contours L0 L1 L2 L3 L4 | L3 L4 L9 L10 L11
sketch "Sketch22" plane through (0, 39.9217, 0) normal (0, -1, 0) x (1, 0, 0)
  line L0 (5.2733, 63.5) -> (-4.8867, 63.5)
  line L1 (-4.8867, 63.5) -> (-4.8867, 43.18)
  line L2 (-4.8867, 43.18) -> (5.2733, 43.18)
  line L3 (5.2733, 43.18) -> (5.2733, 63.5)
  line L4 (-3.0988, 46.9504) -> (-3.1539, 51.2681)
  line L5 (-3.1539, 51.2681) -> (3.0833, 51.308)
  line L6 (3.0833, 51.308) -> (3.0833, 46.99)
  line L7 (3.0833, 46.99) -> (3.11, 44.45)
  line L8 (3.11, 44.45) -> (-3.0988, 44.45)
  line L9 (-3.0988, 44.45) -> (-3.0988, 46.9504)
  line L10 (3.0833, 51.308) -> (4.3533, 51.308)
  line L11 (3.11, 44.45) -> (4.3036, 44.4626)
  line L12 (4.3036, 44.4626) -> (4.3533, 51.308)
  line L13 (-3.1539, 51.2681) -> (-4.4239, 51.2681)
  line L14 (-4.4239, 51.2681) -> (-4.4239, 44.4568)
  line L15 (-4.4239, 44.4568) -> (-3.0988, 44.45)
  dimension "d81" = 1.27
  dimension "d82" = 1.27
extrude "Extrude23" cut 1 faces at (1.8866, 5.7066, 43.18) along direction (0, 0, -1) blind 12.7
extrude "Extrude24" cut 1 faces at (1.8866, 5.7066, 30.48) along direction (0, 0, -1) blind 5.08
sketch "Sketch23" plane through (0, 0, 63.5) normal (0, 0, 1) x (1, 0, 0)
  line L0 (3.0966, 43.0743) -> (3.0966, 41.3657)
  line L1 (3.0966, 41.3657) -> (-3.0988, 41.3657)
  line L2 (-3.0988, 41.3657) -> (-3.0988, 43.0743)
  line L3 (-3.0988, 43.0743) -> (3.0966, 43.0743)
  line L4 (17.7871, 20.3792) -> (17.7871, 25.4592)
  line L5 (17.7871, 25.4592) -> (22.8671, 25.4592)
  line L6 (22.8671, 25.4592) -> (22.8671, 20.3792)
  line L7 (22.8671, 20.3792) -> (17.7871, 20.3792)
  line L8 (-2.5485, -40.6814) -> (-2.5485, -35.3439)
  line L9 (-2.5485, -35.3439) -> (2.5315, -35.3439)
  line L10 (2.5315, -35.3439) -> (2.5315, -40.6814)
  line L11 (2.5315, -40.6814) -> (-2.5485, -40.6814)
  line L12 (-22.7415, 20.3792) -> (-22.7415, 25.4592)
  line L13 (-22.7415, 25.4592) -> (-17.6615, 25.4592)
  line L14 (-17.6615, 25.4592) -> (-17.6615, 20.3792)
  line L15 (-17.6615, 20.3792) -> (-22.7415, 20.3792)
  arc A0 (-31.4879, -5.6993) -> (-31.3557, 6.9834) centre (-31.7467, 0.6454) ccw
  ellipse E0 centre (0, 0) end of major axis (0, 44.45) minor radius 31.75 (-31.4879, -5.6993) -> (31.4886, -5.6926) ccw
  arc A1 (31.355, 6.9901) -> (31.4886, -5.6926) centre (31.7466, 0.6522) ccw
  ellipse E1 centre (0, 0) end of major axis (0, 44.45) minor radius 31.75 (31.355, 6.9901) -> (-31.3557, 6.9834) ccw
  line L16 (7.6088, -16.0819) -> (16.3223, -16.0922)
  line L17 (16.3223, -16.0922) -> (16.3223, -33.833)
  line L18 (16.3223, -33.833) -> (2.3267, -33.8557)
  line L19 (2.3267, -33.8557) -> (-13.4085, -33.833)
  line L20 (-13.4085, -33.833) -> (-15.9357, -33.833)
  line L21 (-15.9357, -33.833) -> (-15.9357, -16.0922)
  line L22 (-15.9357, -16.0922) -> (-13.3958, -16.0922)
  line L23 (-13.3958, -16.0922) -> (-13.3957, -16.053)
  line L24 (-13.3957, -16.053) -> (-7.8668, -16.061)
  line L25 (-7.8668, -16.061) -> (-7.8564, -8.8494)
  line L26 (-7.8564, -8.8494) -> (-10.0299, -8.8463)
  line L27 (-10.0299, -8.8463) -> (-12.5699, -8.9534)
  line L28 (-12.5699, -8.9534) -> (-12.5699, -8.6333)
  line L29 (-12.5699, -8.6333) -> (-15.1099, -8.6009)
  line L30 (-15.1099, -8.6009) -> (-15.1099, 9.1877)
  arc A2 (-15.2005, 9.3115) -> (-15.1099, 9.1877) centre (-10.0299, 12.9977) ccw
  arc A3 (-15.1099, 16.9304) -> (-15.2005, 9.3115) centre (-15.1099, 13.1204) ccw
  line L31 (-15.1099, 16.9304) -> (-15.1099, 34.8417)
  line L32 (-15.1099, 34.8417) -> (-4.8867, 34.8417)
  line L33 (-4.8867, 34.8417) -> (-4.8867, 39.9217)
  line L34 (-4.8867, 39.9217) -> (5.2733, 39.9217)
  line L35 (5.2733, 39.9217) -> (5.2733, 34.8417)
  line L36 (5.2733, 34.8417) -> (15.4965, 34.8417)
  line L37 (15.4965, 34.8417) -> (15.4965, 16.7945)
  arc A4 (15.4965, 9.1715) -> (15.4965, 16.7945) centre (15.4965, 12.983) ccw
  line L38 (15.4965, 9.1715) -> (15.4965, -8.992)
  line L39 (15.4965, -8.992) -> (12.9565, -8.9595)
  line L40 (12.9565, -8.9595) -> (12.9565, -8.992)
  line L41 (12.9565, -8.992) -> (10.4165, -8.8757)
  line L42 (10.4165, -8.8757) -> (7.6191, -8.8717)
  line L43 (7.6191, -8.8717) -> (7.6088, -16.0819)
extrude "Extrude25" add sketch "Sketch23" against normal blind 2.54 contours L12 L13 L14 L15
sketch "Sketch24" plane through (0, 0, 63.5) normal (0, 0, 1) x (1, 0, 0)
  line L0 (3.0966, 43.0743) -> (3.0966, 41.3657)
  line L1 (3.0966, 41.3657) -> (-3.0988, 41.3657)
  line L2 (-3.0988, 41.3657) -> (-3.0988, 43.0743)
  line L3 (-3.0988, 43.0743) -> (3.0966, 43.0743)
  line L4 (17.7871, 20.3792) -> (17.7871, 25.4592)
  line L5 (17.7871, 25.4592) -> (22.8671, 25.4592)
  line L6 (22.8671, 25.4592) -> (22.8671, 20.3792)
  line L7 (22.8671, 20.3792) -> (17.7871, 20.3792)
  line L8 (-2.5485, -40.6814) -> (-2.5485, -35.3439)
  line L9 (-2.5485, -35.3439) -> (2.5315, -35.3439)
  line L10 (2.5315, -35.3439) -> (2.5315, -40.6814)
  line L11 (2.5315, -40.6814) -> (-2.5485, -40.6814)
  arc A0 (-31.4879, -5.6993) -> (-31.3557, 6.9834) centre (-31.7467, 0.6454) ccw
  ellipse E0 centre (0, 0) end of major axis (0, 44.45) minor radius 31.75 (-31.4879, -5.6993) -> (31.4886, -5.6926) ccw
  arc A1 (31.355, 6.9901) -> (31.4886, -5.6926) centre (31.7466, 0.6522) ccw
  ellipse E1 centre (0, 0) end of major axis (0, 44.45) minor radius 31.75 (31.355, 6.9901) -> (-31.3557, 6.9834) ccw
  line L12 (7.6088, -16.0819) -> (16.3223, -16.0922)
  line L13 (16.3223, -16.0922) -> (16.3223, -33.833)
  line L14 (16.3223, -33.833) -> (2.3267, -33.8557)
  line L15 (2.3267, -33.8557) -> (-13.4085, -33.833)
  line L16 (-13.4085, -33.833) -> (-15.9357, -33.833)
  line L17 (-15.9357, -33.833) -> (-15.9357, -16.0922)
  line L18 (-15.9357, -16.0922) -> (-13.3958, -16.0922)
  line L19 (-13.3958, -16.0922) -> (-13.3957, -16.053)
  line L20 (-13.3957, -16.053) -> (-7.8668, -16.061)
  line L21 (-7.8668, -16.061) -> (-7.8564, -8.8494)
  line L22 (-7.8564, -8.8494) -> (-10.0299, -8.8463)
  line L23 (-10.0299, -8.8463) -> (-12.5699, -8.9534)
  line L24 (-12.5699, -8.9534) -> (-12.5699, -8.6333)
  line L25 (-12.5699, -8.6333) -> (-15.1099, -8.6009)
  line L26 (-15.1099, -8.6009) -> (-15.1099, 9.1877)
  arc A2 (-15.2005, 9.3115) -> (-15.1099, 9.1877) centre (-10.0299, 12.9977) ccw
  arc A3 (-15.1099, 16.9304) -> (-15.2005, 9.3115) centre (-15.1099, 13.1204) ccw
  line L27 (-15.1099, 16.9304) -> (-15.1099, 34.8417)
  line L28 (-15.1099, 34.8417) -> (-4.8867, 34.8417)
  line L29 (-4.8867, 34.8417) -> (-4.8867, 39.9217)
  line L30 (-4.8867, 39.9217) -> (5.2733, 39.9217)
  line L31 (5.2733, 39.9217) -> (5.2733, 34.8417)
  line L32 (5.2733, 34.8417) -> (15.4965, 34.8417)
  line L33 (15.4965, 34.8417) -> (15.4965, 16.7945)
  arc A4 (15.4965, 9.1715) -> (15.4965, 16.7945) centre (15.4965, 12.983) ccw
  line L34 (15.4965, 9.1715) -> (15.4965, -8.992)
  line L35 (15.4965, -8.992) -> (12.9565, -8.9595)
  line L36 (12.9565, -8.9595) -> (12.9565, -8.992)
  line L37 (12.9565, -8.992) -> (10.4165, -8.8757)
  line L38 (10.4165, -8.8757) -> (7.6191, -8.8717)
  line L39 (7.6191, -8.8717) -> (7.6088, -16.0819)
  line L40 (20.3271, 22.8395) -> (-20.3538, 22.8395)
  circle A5 centre (-20.3538, 22.8395) radius 2.5
  dimension "d89" = 5
  measures "d89" diameter of A5
extrude "Extrude26" cut sketch "Sketch24" against normal blind 7 contours A5
extrude "Extrude27" add 1 faces at (21.1738, 22.0725, 58.42) along direction (0, 0, 1) blind 5.08
sketch "Sketch25" plane through (0, 0, 63.5) normal (0, 0, 1) x (1, 0, 0)
  circle A0 centre (-20.3538, 22.8395) radius 2.5
  line L0 (3.0966, 43.0743) -> (3.0966, 41.3657)
  line L1 (3.0966, 41.3657) -> (-3.0988, 41.3657)
  line L2 (-3.0988, 41.3657) -> (-3.0988, 43.0743)
  line L3 (-3.0988, 43.0743) -> (3.0966, 43.0743)
  line L4 (-2.5485, -40.6814) -> (-2.5485, -35.3439)
  line L5 (-2.5485, -35.3439) -> (2.5315, -35.3439)
  line L6 (2.5315, -35.3439) -> (2.5315, -40.6814)
  line L7 (2.5315, -40.6814) -> (-2.5485, -40.6814)
  arc A1 (-31.4879, -5.6993) -> (-31.3557, 6.9834) centre (-31.7467, 0.6454) ccw
  ellipse E0 centre (0, 0) end of major axis (0, 44.45) minor radius 31.75 (-31.4879, -5.6993) -> (31.4886, -5.6926) ccw
  arc A2 (31.355, 6.9901) -> (31.4886, -5.6926) centre (31.7466, 0.6522) ccw
  ellipse E1 centre (0, 0) end of major axis (0, 44.45) minor radius 31.75 (31.355, 6.9901) -> (-31.3557, 6.9834) ccw
  line L8 (7.6088, -16.0819) -> (16.3223, -16.0922)
  line L9 (16.3223, -16.0922) -> (16.3223, -33.833)
  line L10 (16.3223, -33.833) -> (2.3267, -33.8557)
  line L11 (2.3267, -33.8557) -> (-13.4085, -33.833)
  line L12 (-13.4085, -33.833) -> (-15.9357, -33.833)
  line L13 (-15.9357, -33.833) -> (-15.9357, -16.0922)
  line L14 (-15.9357, -16.0922) -> (-13.3958, -16.0922)
  line L15 (-13.3958, -16.0922) -> (-13.3957, -16.053)
  line L16 (-13.3957, -16.053) -> (-7.8668, -16.061)
  line L17 (-7.8668, -16.061) -> (-7.8564, -8.8494)
  line L18 (-7.8564, -8.8494) -> (-10.0299, -8.8463)
  line L19 (-10.0299, -8.8463) -> (-12.5699, -8.9534)
  line L20 (-12.5699, -8.9534) -> (-12.5699, -8.6333)
  line L21 (-12.5699, -8.6333) -> (-15.1099, -8.6009)
  line L22 (-15.1099, -8.6009) -> (-15.1099, 9.1877)
  arc A3 (-15.2005, 9.3115) -> (-15.1099, 9.1877) centre (-10.0299, 12.9977) ccw
  arc A4 (-15.1099, 16.9304) -> (-15.2005, 9.3115) centre (-15.1099, 13.1204) ccw
  line L23 (-15.1099, 16.9304) -> (-15.1099, 34.8417)
  line L24 (-15.1099, 34.8417) -> (-4.8867, 34.8417)
  line L25 (-4.8867, 34.8417) -> (-4.8867, 39.9217)
  line L26 (-4.8867, 39.9217) -> (5.2733, 39.9217)
  line L27 (5.2733, 39.9217) -> (5.2733, 34.8417)
  line L28 (5.2733, 34.8417) -> (15.4965, 34.8417)
  line L29 (15.4965, 34.8417) -> (15.4965, 16.7945)
  arc A5 (15.4965, 9.1715) -> (15.4965, 16.7945) centre (15.4965, 12.983) ccw
  line L30 (15.4965, 9.1715) -> (15.4965, -8.992)
  line L31 (15.4965, -8.992) -> (12.9565, -8.9595)
  line L32 (12.9565, -8.9595) -> (12.9565, -8.992)
  line L33 (12.9565, -8.992) -> (10.4165, -8.8757)
  line L34 (10.4165, -8.8757) -> (7.6191, -8.8717)
  line L35 (7.6191, -8.8717) -> (7.6088, -16.0819)
  line L36 (-20.3538, 22.8395) -> (20.1358, 22.8395)
  circle A6 centre (20.1358, 22.8395) radius 2.5
  circle A7 centre (-20.3538, 22.8395) radius 3.5
  dimension "d94" = 5
  dimension "d95" = 7
  measures "d94" diameter of A6
  measures "d95" diameter of A7
extrude "Extrude28" cut sketch "Sketch25" against normal blind 7 contours A7
sketch "Sketch26" plane through (0, 0, 63.5) normal (0, 0, 1) x (1, 0, 0)
  circle A0 centre (-20.3538, 22.8395) radius 3.5
  line L0 (3.0966, 43.0743) -> (3.0966, 41.3657)
  line L1 (3.0966, 41.3657) -> (-3.0988, 41.3657)
  line L2 (-3.0988, 41.3657) -> (-3.0988, 43.0743)
  line L3 (-3.0988, 43.0743) -> (3.0966, 43.0743)
  line L4 (-2.5485, -40.6814) -> (-2.5485, -35.3439)
  line L5 (-2.5485, -35.3439) -> (2.5315, -35.3439)
  line L6 (2.5315, -35.3439) -> (2.5315, -40.6814)
  line L7 (2.5315, -40.6814) -> (-2.5485, -40.6814)
  arc A1 (-31.4879, -5.6993) -> (-31.3557, 6.9834) centre (-31.7467, 0.6454) ccw
  ellipse E0 centre (0, 0) end of major axis (0, 44.45) minor radius 31.75 (-31.4879, -5.6993) -> (31.4886, -5.6926) ccw
  arc A2 (31.355, 6.9901) -> (31.4886, -5.6926) centre (31.7466, 0.6522) ccw
  ellipse E1 centre (0, 0) end of major axis (0, 44.45) minor radius 31.75 (31.355, 6.9901) -> (-31.3557, 6.9834) ccw
  line L8 (7.6088, -16.0819) -> (16.3223, -16.0922)
  line L9 (16.3223, -16.0922) -> (16.3223, -33.833)
  line L10 (16.3223, -33.833) -> (2.3267, -33.8557)
  line L11 (2.3267, -33.8557) -> (-13.4085, -33.833)
  line L12 (-13.4085, -33.833) -> (-15.9357, -33.833)
  line L13 (-15.9357, -33.833) -> (-15.9357, -16.0922)
  line L14 (-15.9357, -16.0922) -> (-13.3958, -16.0922)
  line L15 (-13.3958, -16.0922) -> (-13.3957, -16.053)
  line L16 (-13.3957, -16.053) -> (-7.8668, -16.061)
  line L17 (-7.8668, -16.061) -> (-7.8564, -8.8494)
  line L18 (-7.8564, -8.8494) -> (-10.0299, -8.8463)
  line L19 (-10.0299, -8.8463) -> (-12.5699, -8.9534)
  line L20 (-12.5699, -8.9534) -> (-12.5699, -8.6333)
  line L21 (-12.5699, -8.6333) -> (-15.1099, -8.6009)
  line L22 (-15.1099, -8.6009) -> (-15.1099, 9.1877)
  arc A3 (-15.2005, 9.3115) -> (-15.1099, 9.1877) centre (-10.0299, 12.9977) ccw
  arc A4 (-15.1099, 16.9304) -> (-15.2005, 9.3115) centre (-15.1099, 13.1204) ccw
  line L23 (-15.1099, 16.9304) -> (-15.1099, 34.8417)
  line L24 (-15.1099, 34.8417) -> (-4.8867, 34.8417)
  line L25 (-4.8867, 34.8417) -> (-4.8867, 39.9217)
  line L26 (-4.8867, 39.9217) -> (5.2733, 39.9217)
  line L27 (5.2733, 39.9217) -> (5.2733, 34.8417)
  line L28 (5.2733, 34.8417) -> (15.4965, 34.8417)
  line L29 (15.4965, 34.8417) -> (15.4965, 16.7945)
  arc A5 (15.4965, 9.1715) -> (15.4965, 16.7945) centre (15.4965, 12.983) ccw
  line L30 (15.4965, 9.1715) -> (15.4965, -8.992)
  line L31 (15.4965, -8.992) -> (12.9565, -8.9595)
  line L32 (12.9565, -8.9595) -> (12.9565, -8.992)
  line L33 (12.9565, -8.992) -> (10.4165, -8.8757)
  line L34 (10.4165, -8.8757) -> (7.6191, -8.8717)
  line L35 (7.6191, -8.8717) -> (7.6088, -16.0819)
  line L36 (-20.3538, 22.8395) -> (15.4965, 22.871)
  line L37 (15.4965, 22.871) -> (20.7289, 22.871)
  circle A6 centre (20.7289, 22.871) radius 3.5
  dimension "d98" = 5.2324
  dimension "d99" = 7
  measures "d98" distance of E0.centre
  measures "d99" diameter of A6
extrude "Extrude29" cut sketch "Sketch26" against normal blind 7 contours A6